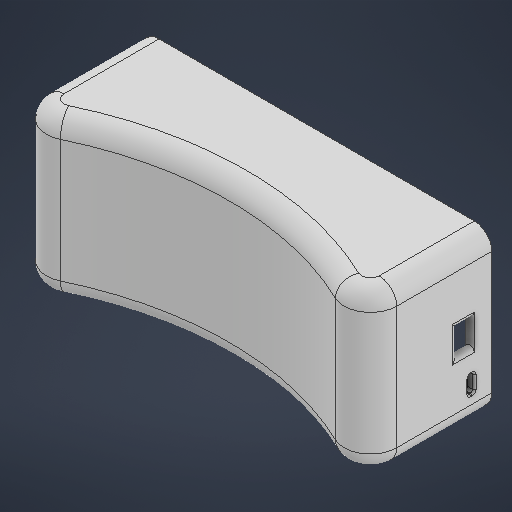
# Autodesk Inventor part: BatPackCase
Saved by Autodesk Inventor 2025 (Build 290162010, 162A)
## iProperties
Created: 2024-05-30
Part Number: BatPackCase
Material: Generic
Document SubType Name: Modeling
Designer: techn
Density: 1 g/cm^3
Appearance: Default
Author: techn
## iProperties of the stored document BatPackCase_3DPrint.ipt
Created: 2024-06-19
Part Number: BatPackCase_3DPrint
Material: Generic
Document SubType Name: Modeling
Designer: techn
Density: 1 g/cm^3
Appearance: Default
Author: techn
Autodesk Inventor part; units mm, degrees
ref_plane "YZ Plane" through (0, 0, 0) normal (1, 0, 0) x (0, 1, 0)
ref_plane "XZ Plane" through (0, 0, 0) normal (0, 1, 0) x (-1, 0, 0)
ref_plane "XY Plane" through (0, 0, 0) normal (0, 0, 1) x (1, 0, 0)
sketch "Sketch1" plane through (0, 0, 0) normal (0, 0, 1) x (1, 0, 0)
  line L0 (0, 0) -> (200, 0)
  line L1 (200, 0) -> (200, 90)
  line L2 (200, 90) -> (0, 90)
  line L3 (0, 90) -> (0, 0)
  dimension "d0" = 200
  dimension "d1" = 90
  constraints: 8 end point, 2 parallel, 1 horizontal, 1 perpendicular
  measures "d0" distance of L2.end L1.end
  measures "d1" distance of L1.end L0.end
extrude "Extrusion1" add sketch "Sketch1" against normal blind 80
sketch "Sketch2" plane through (0, 90, 0) normal (0, 1, 0) x (1, 0, 0)
  line L0 (200, 0) -> (0, 0) projected
  line L1 (200, 0) -> (200, 80) projected
  line L2 (0, 80) -> (200, 80) projected
  line L3 (0, 0) -> (0, 80) projected
  circle A0 centre (100, 0) radius 30
  arc A1 (200, 0) -> (0, 0) centre (100, -151.6667) ccw
  dimension "d4" = 60
  constraints: 2 centre point, 2 point on circle, 1 midpoint
  measures "d4" diameter of A0
extrude "Extrusion2" cut sketch "Sketch2" against normal blind 100 contours L0 A0 A1 | L0 A0 | A0 L0 A1 picked at (94.9216, 15.5737)
fillet "Fillet1" radius 15 2 edges at (200, 45, 0) (0, 45, 0)
sketch "Sketch3" plane through (200, 0, -80) normal (1, 0, 0) x (0, 0, -1)
  line L0 (-80, 0) -> (-80, 90) projected
  line L1 (-80, 0) -> (0, 0) projected
  line L2 (0, 90) -> (0, 0) projected
  line L3 (-80, 90) -> (0, 90) projected
  line L4 (-12, 25) -> (-11.3, 25)
  line L5 (-10, 23.7) -> (-10, 16.3)
  line L6 (-11.3, 15) -> (-12, 15)
  line L7 (-13.3, 16.3) -> (-13.3, 23.7)
  arc A0 (-12, 25) -> (-13.3, 23.7) centre (-12, 23.7) ccw
  arc A1 (-10, 23.7) -> (-11.3, 25) centre (-11.3, 23.7) ccw
  arc A2 (-11.3, 15) -> (-10, 16.3) centre (-11.3, 16.3) ccw
  arc A3 (-13.3, 16.3) -> (-12, 15) centre (-12, 16.3) ccw
  point P0 (-10, 15)
  point P1 (-10, 25)
  point P2 (-13.3, 15)
  point P3 (-11.65, 15)
  dimension "d8" = 3.3
  dimension "d9" = 10
  dimension "d10" = 1.3
  dimension "d11" = 10
  dimension "d12" = 15
  constraints: 8 end point, 8 point on circle, 8 tangent, 6 point on line, 4 centre point, 3 equal radius, 2 parallel, 1 horizontal, 1 midpoint, 1 perpendicular
  measures "d8" distance of point (-10, 15) point (-13.3, 15)
  measures "d9" distance of point (-10, 25) point (-10, 15)
  measures "d10" radius of A0
  measures "d11" distance between parallel lines of L2 L5
  measures "d12" distance from line of L1 point (-11.65, 15)
fillet "Fillet3" radius 10 10 edges at (7.0077, 0, -12.9892) (0, 0, -52.8413) (192.9923, 0, -12.9892) (200, 0, -52.8413) (100, 0, -30) (192.9923, 90, -12.9892) (200, 90, -52.8413) (7.0077, 90, -12.9892) (0, 90, -52.8413) (100, 90, -30)
shell "Shell2" thickness 5 removed faces 1 at (130, 30, -80)
extrude "Extrusion4" cut sketch "Sketch3" against normal blind 100 contours L4 A1 L5 A2 L6 A3 L7 A0
fillet "Fillet4" radius 1 16 edges at (200, 24.6192, -67.0808) (200, 25, -68.35) (200, 24.6192, -69.6192) (200, 20, -70) (200, 15.3808, -69.6192) (200, 15, -68.35) (200, 15.3808, -67.0808) (200, 20, -66.7) (195, 15.3808, -67.0808) (195, 15, -68.35) (195, 15.3808, -69.6192) (195, 20, -70) (195, 24.6192, -69.6192) (195, 25, -68.35) (195, 24.6192, -67.0808) (195, 20, -66.7)
sketch "Sketch6" plane through (200, 10, -25.6826) normal (1, 0, 0) x (0, 0, -1)
  line L0 (0, 70) -> (54.3174, 70) projected
  line L1 (0, 0) -> (0, 70) projected
  line L2 (54.3174, 0) -> (0, 0) projected
  line L3 (54.3174, 70) -> (54.3174, 0) projected
  arc A0 (42.3174, 16) -> (40.0174, 13.7) centre (42.3174, 13.7) ccw projected
  line L4 (43.0174, 16) -> (42.3174, 16) projected
  arc A1 (45.3174, 13.7) -> (43.0174, 16) centre (43.0174, 13.7) ccw projected
  line L5 (45.3174, 6.3) -> (45.3174, 13.7) projected
  arc A2 (43.0174, 4) -> (45.3174, 6.3) centre (43.0174, 6.3) ccw projected
  line L6 (42.3174, 4) -> (43.0174, 4) projected
  arc A3 (40.0174, 6.3) -> (42.3174, 4) centre (42.3174, 6.3) ccw projected
  line L7 (40.0174, 13.7) -> (40.0174, 6.3) projected
  line L8 (44.3174, 42.5) -> (34.3174, 42.5)
  line L9 (34.3174, 42.5) -> (34.3174, 27.5)
  line L10 (34.3174, 27.5) -> (44.3174, 27.5)
  line L11 (44.3174, 27.5) -> (44.3174, 42.5)
  point P0 (-25.6826, -10)
  point P1 (44.3174, 35)
  point P2 (54.3174, 35)
  dimension "d32" = 10
  dimension "d33" = 15
  dimension "d34" = 10
  constraints: 8 end point, 2 midpoint, 2 parallel, 1 horizontal, 1 horizontal alignment, 1 perpendicular
  measures "d32" distance of L10.end L9.end
  measures "d33" distance of L9.end L8.end
  measures "d34" distance between parallel lines of L3 L11
extrude "Extrusion7" cut sketch "Sketch6" against normal blind 5 contours L11 L10 L9 L8
sketch "Sketch7" plane through (0, 10, -80) normal (-1, 0, 0) x (0, 0, 1)
  line L0 (0, 70) -> (54.3174, 70) projected
  line L1 (0, 0) -> (0, 70) projected
  line L2 (54.3174, 0) -> (0, 0) projected
  line L3 (54.3174, 70) -> (54.3174, 0) projected
  line L4 (10, 42.5) -> (20, 42.5)
  line L5 (20, 42.5) -> (20, 27.5)
  line L6 (20, 27.5) -> (10, 27.5)
  line L7 (10, 27.5) -> (10, 42.5)
  point P0 (80, -10)
  point P1 (10, 35)
  point P2 (0, 35)
  dimension "d37" = 10
  dimension "d38" = 15
  dimension "d39" = 10
  constraints: 8 end point, 2 midpoint, 2 parallel, 1 horizontal, 1 horizontal alignment, 1 perpendicular
  measures "d37" distance of L5.end L6.end
  measures "d38" distance of L4.end L5.end
  measures "d39" distance between parallel lines of L1 L7
extrude "Extrusion8" cut sketch "Sketch7" against normal blind 5 contours L4 L5 L6 L7
fillet "Fillet5" radius 2.5 12 edges at (195, 45, -60) (195, 52.5, -65) (195, 37.5, -65) (200, 45, -60) (200, 37.5, -65) (200, 52.5, -65) (0, 45, -60) (5, 45, -60) (5, 52.5, -65) (0, 52.5, -65) (0, 37.5, -65) (5, 37.5, -65)
body "Solid1"
